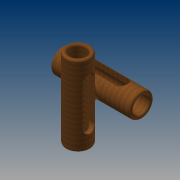
# Autodesk Inventor part: Socket
Saved by Autodesk Inventor 2014 (Build 180170000, 170)
## iProperties
Created: 2021-03-29
Part Number: Socket
Material: Copper, Cast
Document SubType Name: Modeling
Designer: Diptanshu Das
Density: 8.94 g/cm^3
Appearance: Rust
Author: Diptanshu Das
Autodesk Inventor part; units mm, degrees
sketch "Sketch1" plane through (0, 0, 0) normal (0, 0, 1) x (1, 0, 0)
  circle A0 centre (0, 0) radius 30
  circle A1 centre (0, 0) radius 20
  dimension "d0" = 60
  dimension "d1" = 40
  constraints: 2 centre point, 2 coincident
  measures "d0" diameter of A0
  measures "d1" diameter of A1
extrude "Extrusion1" add sketch "Sketch1" along normal blind 200
fillet "Fillet1" radius 5 4 edges at (-20, 0, 200) (-30, 0, 200) (-20, 0, 0) (-30, 0, 0)
ref_plane "Work Plane1" through (30, 0, 0) normal (1, 0, 0) x (0, 1, 0)
sketch "Sketch2" plane through (30, 0, 0) normal (1, 0, 0) x (0, 1, 0)
  line L0 (0, 50) -> (0, 150) construction
  line L1 (-15, 50) -> (-15, 150)
  line L2 (15, 150) -> (15, 50)
  arc A0 (-15, 50) -> (15, 50) centre (0, 50) ccw
  arc A1 (15, 150) -> (-15, 150) centre (0, 150) ccw
  line L3 (25, 0) -> (-25, 0) projected
  point P0 (0, 0)
  point P1 (0, 100)
  dimension "d6" = 100
  dimension "d7" = 15
  dimension "d8" = 100
  constraints: 8 end point, 4 point on circle, 4 tangent, 2 centre point, 1 midpoint, 1 parallel, 1 vertical
  measures "d6" distance of L0.start L0.end
  measures "d7" radius of A0
  measures "d8" distance from line of point (0, 100) L3
extrude "Extrusion2" cut sketch "Sketch2" against normal blind 150
ref_plane "Work Plane2" through (0, 30, 0) normal (0, 1, 0) x (-1, 0, 0)
sketch "Sketch3" plane through (0, 30, 0) normal (0, 1, 0) x (-1, 0, 0)
  circle A0 centre (0, 100) radius 20
  line L0 (-25, 200) -> (25, 200) projected
  point P0 (0, 0)
  dimension "d12" = 40
  dimension "d13" = 100
  constraints: 1 centre point
  measures "d12" diameter of A0
  measures "d13" distance from line of L0 A0.centre
extrude "Extrusion3" add sketch "Sketch3" along normal blind 10 and the other way blind 10
sketch "Sketch4" plane through (0, 0, 0) normal (1, 0, 0) x (0, 1, 0)
  circle A0 centre (60, 100.9967) radius 30
  circle A1 centre (60, 100.9967) radius 20
  line L0 (40, 80) -> (40, 120) projected
  line L1 (30, 5) -> (30, 195) projected
  point P0 (0, 0)
  dimension "d18" = 60
  dimension "d19" = 40
  dimension "d21" = 30
  constraints: 2 centre point, 1 coincident
  measures "d18" diameter of A0
  measures "d19" diameter of A1
  measures "d21" distance from line of L1 A0.centre
extrude "Extrusion4" add sketch "Sketch4" along normal mid plane 200
fillet "Fillet2" radius 5 4 edges at (100, 40, 100.9967) (100, 30, 100.9967) (-100, 40, 100.9967) (-100, 30, 100.9967)
ref_plane "Work Plane3" through (0, 0, 100) normal (0, 0, 1) x (1, 0, 0)
sketch "Sketch5" plane through (0, 0, 100) normal (0, 0, 1) x (1, 0, 0)
  line L0 (-50, 60) -> (50, 60) construction
  line L1 (-50, 45) -> (50, 45)
  line L2 (50, 75) -> (-50, 75)
  arc A0 (-50, 75) -> (-50, 45) centre (-50, 60) ccw
  arc A1 (50, 45) -> (50, 75) centre (50, 60) ccw
  line L3 (-95, 90) -> (95, 90) projected
  line L4 (100, 85) -> (100, 35) projected
  point P0 (0, 0)
  point P1 (0, 60)
  dimension "d26" = 100
  dimension "d27" = 15
  dimension "d28" = 30
  dimension "d29" = 100
  constraints: 8 end point, 4 point on circle, 4 tangent, 2 centre point, 1 horizontal, 1 midpoint, 1 parallel
  measures "d26" distance of L0.start L0.end
  measures "d27" radius of A0
  measures "d28" distance from line of point (0, 60) L3
  measures "d29" distance from line of L4 point (0, 60)
extrude "Extrusion5" cut sketch "Sketch5" along normal mid plane 200
fillet "Fillet3" radius 5 8 edges at (-12.6904, 33.7157, 115.4581) (12.691, 33.7154, 115.4576) (13.3085, 34.5763, 85.0707) (-13.0357, 34.7275, 84.8319) (-19.9938, 30.0041, 100.4985) (-15.1929, 25.8684, 86.9932) (-15.1929, 25.8684, 113.0068) (20, 22.3607, 100.0107)
body "Solid1"
